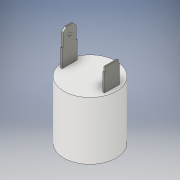
# Autodesk Inventor part: Zündspule
Saved by Autodesk Inventor 2017 (Build 210142000, 142)
## iProperties
Part Number: Zündspule
Material: Generisch
Document SubType Name: Modeling
Designer: David Merges
Density: 1 g/cm^3
Appearance: Weiß
Author: David Merges
Autodesk Inventor part; units mm, degrees
ref_plane "YZ Plane" through (0, 0, 0) normal (1, 0, 0) x (0, 1, 0)
ref_plane "XZ Plane" through (0, 0, 0) normal (0, 1, 0) x (-1, 0, 0)
ref_plane "XY Plane" through (0, 0, 0) normal (0, 0, 1) x (1, 0, 0)
sketch "Skizze1" plane through (0, 0, 0) normal (0, 0, 1) x (1, 0, 0)
  circle A0 centre (0, 0) radius 13.1
  dimension "d0" = 26.2
  constraints: 1 centre point, 1 coincident
  measures "d0" diameter of A0
extrude "Extrusion1" add sketch "Skizze1" along normal blind 29
sketch "Skizze2" plane through (0, 0, 29) normal (0, 0, 1) x (1, 0, 0)
  line L0 (-11, 3.75) -> (-10.2, 3.75)
  line L1 (-10.2, 3.75) -> (-10.2, -3.75)
  line L2 (-10.2, -3.75) -> (-11, -3.75)
  line L3 (-11, -3.75) -> (-11, 3.75)
  line L4 (10.2, 3.75) -> (11, 3.75)
  line L5 (11, 3.75) -> (11, -3.75)
  line L6 (11, -3.75) -> (10.2, -3.75)
  line L7 (10.2, -3.75) -> (10.2, 3.75)
  line L8 (10.2, 0) -> (-10.2, 0) construction
  point P0 (0, 0)
  point P1 (0, 0)
  dimension "d3" = 7.5
  dimension "d4" = 0.8
  dimension "d6" = 22
  constraints: 18 end point, 4 parallel, 3 horizontal, 3 midpoint, 2 equal length, 2 perpendicular, 1 coincident
  measures "d3" distance of L2.end L0.start
  measures "d4" distance of L0.start L0.end
  measures "d6" distance between parallel lines of L5 L3
sketch "Skizze3" plane through (0, 0, 0) normal (0, 1, 0) x (-1, 0, 0)
  line L0 (13.1, 29) -> (-13.1, 29) projected
  line L1 (-13.1, 0) -> (13.1, 0) projected
  line L2 (-13.1, 0) -> (-13.1, 29) projected
  line L3 (13.1, 0) -> (13.1, 29) projected
  point P0 (0, 0)
  dimension "d7" = 29
  measures "d7" distance of L2.start L2.end
extrude "Extrusion2" add sketch "Skizze2" along normal blind 17
sketch "Skizze4" plane through (11, -3.75, 29) normal (1, 0, 0) x (0, 0, -1)
  line L0 (0, 7.5) -> (0, 0) projected
  line L1 (0, 7.5) -> (-17, 7.5) construction
  line L2 (-17, 0) -> (-17, 7.5) construction
  line L3 (0, 0) -> (-17, 0) construction
  line L4 (0, 0) -> (-17, 0) construction
  line L5 (-9, 0) -> (-9, 0.55)
  line L6 (-9, 0.55) -> (-15.5, 0.55)
  line L7 (-15.5, 0.55) -> (-17, 2.05)
  line L8 (-17, 5.45) -> (-15.5, 6.95)
  line L9 (-15.5, 6.95) -> (-9, 6.95)
  line L10 (-9, 6.95) -> (-9, 7.5)
  line L11 (0, 7.5) -> (-17, 7.5) construction
  circle A0 centre (-13, 3.75) radius 0.9
  line L12 (-13, 3.75) -> (-17, 3.75) construction
  line L13 (-17, 0) -> (-17, 7.5) construction
  line L14 (-17, 0) -> (-17, 7.5) construction
  line L15 (-9, 0) -> (-17, 0)
  line L16 (-17, 2.05) -> (-17, 0)
  line L17 (-17, 5.45) -> (-17, 7.5)
  line L18 (-9, 7.5) -> (-17, 7.5)
  point P0 (29, 3.75)
  dimension "d10" = 45
  dimension "d11" = 45
  dimension "d12" = 6.4
  dimension "d13" = 8
  dimension "d14" = 1.5
  dimension "d15" = 1.8
  dimension "d16" = 4
  constraints: 22 end point, 6 point on line, 3 perpendicular, 2 collinear, 2 equal length, 1 centre point, 1 horizontal, 1 midpoint, 1 parallel, 1 vertical
  measures "d10" angle of L6 L7
  measures "d11" angle of L8 L9
  measures "d12" distance between parallel lines of L6 L9
  measures "d13" distance between parallel lines of L2 L5
  measures "d14" distance from line of L7.end L6
  measures "d15" diameter of A0
  measures "d16" distance of L12.start L12.end
extrude "Extrusion3" cut sketch "Skizze4" against normal through all
sketch "Skizze5" plane through (0, 0, 0) normal (0, 0, -1) x (-1, 0, 0)
  line L0 (-3, 2) -> (3, 2)
  line L1 (3, 2) -> (3, -2)
  line L2 (3, -2) -> (-3, -2)
  line L3 (-3, -2) -> (-3, 2)
  line L4 (3, -2) -> (-3, 2) construction
  point P0 (0, 0)
  point P1 (0, 0)
  dimension "d19" = 6
  dimension "d20" = 4
  constraints: 10 end point, 2 parallel, 1 coincident, 1 horizontal, 1 midpoint, 1 perpendicular
  measures "d19" distance of L1.end L2.end
  measures "d20" distance of L0.end L1.end
extrude "Extrusion4" cut sketch "Skizze5" against normal blind 0.2
sketch "Skizze6" plane through (11, -3.75, 29) normal (1, 0, 0) x (0, 0, -1)
  line L0 (-17, 7.5187) -> (-11, 7.5187)
  line L1 (-11, 7.5187) -> (-11, -0.0187)
  line L2 (-11, -0.0187) -> (-17, -0.0187)
  line L3 (-17, -0.0187) -> (-17, 7.5187)
  line L4 (-17, 2.05) -> (-17, 5.45) projected
  point P0 (29, 3.75)
  point P1 (-17, 3.75)
  dimension "d23" = 6
  constraints: 8 end point, 2 midpoint, 2 parallel, 1 horizontal, 1 perpendicular
  measures "d23" distance of L2.end L1.end
extrude "Extrusion5" cut sketch "Skizze6" against normal blind 1
equation "\"d11\" = d10"
